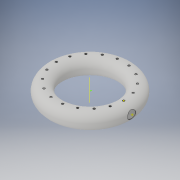
# Autodesk Inventor part: Burner
Saved by Autodesk Inventor 2019 (Build 230136000, 136)
## iProperties
Created: 2019-12-13
Part Number: Burner
Material: Generic
Document SubType Name: Modeling
Designer: Administrator
Density: 1 g/cm^3
Appearance: Default
Author: Administrator
Autodesk Inventor part; units mm, degrees
sketch "Sketch3" plane through (0, 0, 0) normal (0, 0, 1) x (1, 0, 0)
  circle A0 centre (0, 0) radius 25.4
  circle A1 centre (0, 0) radius 24.13
  line L0 (0, 0) -> (-102.87, 0) construction
  line L1 (-102.87, 0) -> (-102.87, 127) construction
  line L2 (0, 0) -> (-25.4, 0) construction
  line L3 (25.4, 0) -> (25.4, 25.4)
  dimension "d3" = 50.8
  dimension "d4" = 48.26
  dimension "d10" = 102.87
  dimension "d11" = 127
  constraints: 8 end point, 2 centre point, 2 coincident, 2 point on circle, 2 vertical, 1 horizontal, 1 point on line, 1 tangent
  measures "d3" diameter of A0
  measures "d4" diameter of A1
  measures "d10" distance of L0.start L0.end
  measures "d11" distance of L0.end L1.end
revolve "Revolution1" add sketch "Sketch3" angle 360 about axis through (-102.87, 0, 0) along (0, 1, 0)
ref_plane "Work Plane4" through (-102.87, 0, 0) normal (0, -1, 0) x (1, 0, 0)
ref_plane "Work Plane6" through (-102.87, 0, 0) normal (0, -1, 0) x (1, 0, 0)
sketch "Sketch12" plane through (-102.87, 0, 0) normal (0, -1, 0) x (1, 0, 0)
  line L0 (0, 0) -> (0, -3.9825)
  point P0 (102.87, 0)
  constraints: 2 end point, 1 vertical
sketch3d "3D Sketch7"
ref_plane "Work Plane7" through (-102.87, 25.4, 0) normal (0, -1, 0) x (1, 0, 0)
sketch "Sketch13" plane through (-102.87, 25.4, 0) normal (0, -1, 0) x (1, 0, 0)
  line L0 (51.435, 0) -> (102.87, 0) construction
  circle A0 centre (102.87, 0) radius 3.175
  dimension "d18" = 6.35
  constraints: 2 end point, 1 centre point, 1 coincident, 1 horizontal
  measures "d18" diameter of A0
extrude "Extrusion1" cut sketch "Sketch13" along normal blind 25.4
pattern_circular "Circular Pattern1" count 18 over 360 about axis through (-102.87, 0, 0) along (0, -1, 0) of "Extrusion1"
sketch "Sketch14" plane through (-102.87, 25.4, 0) normal (0, -1, 0) x (1, 0, 0)
  point P0 (102.87, 0)
ref_plane "Work Plane8" through (25.4, 25.4, 0) normal (0, 1, 0) x (-1, 0, 0)
sketch "Sketch15" plane through (25.4, 25.4, 0) normal (0, 1, 0) x (-1, 0, 0)
  line L0 (0, 0) -> (0, -12.7)
  circle A0 centre (128.27, 0) radius 128.27 projected
  point P0 (25.4, 0)
  dimension "d26" = 12.7
  constraints: 2 end point, 1 tangent, 1 vertical
  measures "d26" distance of L0.start L0.end
ref_plane "Work Plane9" through (25.4, 0, 0) normal (-1, 0, 0) x (0, 1, 0)
sketch "Sketch17" plane through (25.4, 0, 0) normal (-1, 0, 0) x (0, 1, 0)
  circle A0 centre (0, 0) radius 12.7
  dimension "d29" = 25.4
  constraints: 1 centre point, 1 coincident
  measures "d29" diameter of A0
extrude "Extrusion3" cut sketch "Sketch17" along normal blind 12.7
body "Solid1"
